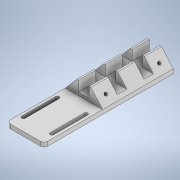
# Autodesk Inventor part: sun2
Saved by Autodesk Inventor 2021 (Build 250183000, 183)
## iProperties
Created: 2021-04-13
Part Number: sun2
Material: 일반
Document SubType Name: Modeling
Designer: Dongyoon
Density: 1 g/cm^3
Appearance: 기본값
Author: Dongyoon
Autodesk Inventor part; units mm, degrees
ref_plane "YZ Plane" through (0, 0, 0) normal (1, 0, 0) x (0, 1, 0)
ref_plane "XZ Plane" through (0, 0, 0) normal (0, 1, 0) x (-1, 0, 0)
ref_plane "XY Plane" through (0, 0, 0) normal (0, 0, 1) x (1, 0, 0)
sketch "스케치1" plane through (0, 0, 0) normal (0, 1, 0) x (-1, 0, 0)
  line L0 (-21.65, 75) -> (21.65, 75)
  line L1 (21.65, 75) -> (21.65, -75)
  line L2 (21.65, -75) -> (-21.65, -75)
  line L3 (-21.65, -75) -> (-21.65, 75)
  line L4 (-21.65, 75) -> (21.65, -75) construction
  line L5 (21.65, 75) -> (-21.65, -75) construction
  line L6 (-21.65, 7) -> (21.65, 7)
  point P0 (0, 0)
  dimension "d0" = 43.3
  dimension "d1" = 150
  dimension "d2" = 68
  constraints: 14 end point, 2 midpoint, 2 parallel, 2 perpendicular, 2 point on line, 1 horizontal
  measures "d0" distance of L1.end L2.end
  measures "d1" distance of L2.end L0.start
  measures "d2" distance between parallel lines of L0 L6
extrude "돌출2" add sketch "스케치1" along normal blind 5 contours L0 L1 L6 L3
extrude "돌출3" add sketch "스케치1" along normal blind 8.5 contours L6 L1 L2 L3
sketch "스케치3" plane through (0, 8.5, 0) normal (0, 1, 0) x (1, 0, 0)
  line L0 (-21.65, -7) -> (21.65, -7) projected
  line L1 (21.65, 75) -> (-21.65, 75) projected
  line L2 (6.1, -7) -> (-6.1, -7)
  line L3 (-6.1, -7) -> (-6.1, 75)
  line L4 (-6.1, 75) -> (6.1, 75)
  line L5 (6.1, 75) -> (6.1, -7)
  line L6 (21.65, -7) -> (21.65, 75) projected
  line L7 (21.65, 75) -> (6.1, 75)
  line L8 (6.1, 75) -> (6.1, -7)
  line L9 (6.1, -7) -> (21.65, -7)
  line L10 (21.65, -7) -> (21.65, 75)
  line L11 (-21.65, 75) -> (-6.1, 75)
  line L12 (-6.1, 75) -> (-6.1, -7)
  line L13 (-6.1, -7) -> (-21.65, -7)
  line L14 (-21.65, -7) -> (-21.65, 75)
  point P0 (0, 0)
  point P1 (-6.1, -7)
  point P2 (6.1, 75)
  dimension "d9" = 12.2
  dimension "d11" = 6.1
  constraints: 24 end point, 6 parallel, 3 horizontal, 3 perpendicular, 2 point on line
  measures "d9" distance between parallel lines of L5 L3
  measures "d11" distance from line of point (0, 0) L5
extrude "돌출4" add sketch "스케치3" along normal blind 12.2 contours L14 L1 L3 L0 | L5 L1 L6 L0
sketch "스케치4" plane through (0, 5, 0) normal (0, 1, 0) x (1, 0, 0)
  line L0 (16.55, -19.1) -> (16.55, -62.7) construction
  line L1 (14.55, -21.1) -> (14.55, -60.7)
  line L2 (18.55, -60.7) -> (18.55, -21.1)
  arc A0 (18.55, -21.1) -> (14.55, -21.1) centre (16.55, -21.1) ccw
  arc A1 (14.55, -60.7) -> (18.55, -60.7) centre (16.55, -60.7) ccw
  line L3 (21.65, -75) -> (21.65, -7) projected
  line L4 (-21.65, -75) -> (21.65, -75) projected
  line L5 (21.65, -7) -> (-21.65, -7) projected
  line L6 (0, -7) -> (0, -75)
  line L7 (-16.55, -19.1) -> (-16.55, -62.7) construction
  line L8 (-14.55, -21.1) -> (-14.55, -60.7)
  line L9 (-18.55, -60.7) -> (-18.55, -21.1)
  arc A2 (-14.55, -21.1) -> (-18.55, -21.1) centre (-16.55, -21.1) ccw
  arc A3 (-18.55, -60.7) -> (-14.55, -60.7) centre (-16.55, -60.7) ccw
  point P0 (0, 0)
  point P1 (16.55, -40.9)
  point P2 (-16.55, -40.9)
  dimension "d14" = 43.6
  dimension "d15" = 3.1
  dimension "d16" = 4
  dimension "d17" = 12.3
  constraints: 18 end point, 12 point on circle, 9 symmetric about line, 4 centre point, 4 point on line, 4 tangent, 3 midpoint, 1 parallel, 1 vertical, 2 other
  measures "d14" distance of L0.start L0.end
  measures "d15" distance between parallel lines of L3 L2
  measures "d16" distance between parallel lines of L2 L1
  measures "d17" distance from line of L4 L0.end
extrude "돌출5" cut sketch "스케치4" against normal through all contours A0 L2 A1 L1 | L8 A3 L9 A2
fillet "모깎기1" radius 4.5 2 edges at (21.65, 2.5, 75) (-21.65, 2.5, 75)
sketch "스케치5" plane through (-21.65, 5, 7) normal (0, 0, 1) x (1, 0, 0)
  line L0 (27.75, 3.5) -> (15.55, 3.5) projected
  line L1 (21.65, 3.5) -> (21.65, 29.9168)
  line L2 (43.3, 0) -> (43.3, 15.7) projected
  line L3 (4.5, 0) -> (38.8, 0) projected
  line L4 (43.3, 15.7) -> (27.75, 15.7)
  line L5 (27.75, 15.7) -> (27.75, 0)
  line L6 (27.75, 0) -> (43.3, 0)
  line L7 (43.3, 0) -> (43.3, 15.7)
  line L8 (43.3, 0) -> (29.75, 15.7)
  line L9 (43.3, 15.7) -> (27.75, 15.7) projected
  line L10 (43.3, -5) -> (38.8, -5) projected
  line L11 (0, 0) -> (0, 15.7)
  line L12 (0, 15.7) -> (15.55, 15.7)
  line L13 (0, 0) -> (0, 15.7)
  line L14 (0, 0) -> (13.55, 15.7)
  point P0 (21.65, -5)
  dimension "d21" = 2
  dimension "d22" = 5
  constraints: 20 end point, 6 symmetric about line, 4 point on line, 2 parallel, 1 horizontal, 1 midpoint, 1 perpendicular, 1 vertical
  measures "d21" distance of L4.end L8.end
  measures "d22" distance from line of L10 L8.start
extrude "돌출6" cut sketch "스케치5" against normal through all contours L8 L4 L2 | L11 L12 L14
sketch "스케치7" plane through (-21.65, 5, -75) normal (-0.7570398, 0.6533688, 0) x (0, 0, 1)
  line L0 (0, 20.7387) -> (82, 20.7387) projected
  line L1 (82, 0) -> (0, 0) projected
  line L2 (82, 20.7387) -> (82, 0) projected
  circle A0 centre (10, 9.7387) radius 1.75
  line L3 (82, 28.2909) -> (82, 0) projected
  line L4 (82, 9.7387) -> (0, 9.7387)
  line L5 (0, 24.5057) -> (0, -3.7852) projected
  line L6 (82, 20.7806) -> (0, 20.7806) projected
  line L7 (41, 20.7806) -> (41, 0)
  circle A1 centre (72, 9.7387) radius 1.75
  dimension "d26" = 3.5
  dimension "d28" = 10
  dimension "d39" = 11
  constraints: 4 end point, 3 point on line, 2 centre point, 2 midpoint, 1 horizontal, 1 symmetric about line, 1 other
  measures "d26" diameter of A0
  measures "d28" distance from line of L5 A0.centre
  measures "d39" distance from line of L0 A0.centre
extrude "돌출7" cut sketch "스케치7" against normal blind 10 contours L4 A0 | A0 L4 | A1 L4 | L4 A1
mirror "미러1" about plane through (0, 0, 0) normal (1, 0, 0) of "돌출7"
sketch "스케치9" plane through (0, 8.5, 0) normal (0, 1, 0) x (1, 0, 0)
  ellipse E0 centre (-15.2871, 3) end of major axis (-15.2871, 1.25) minor radius 1.1434 projected
  ellipse E1 centre (-15.2871, 65) end of major axis (-15.2871, 63.25) minor radius 1.1434 projected
  line L0 (-29.6157, 34) -> (32.1158, 34)
  line L1 (-21.65, -7) -> (-21.65, 75) projected
  line L2 (21.65, 75) -> (21.65, -7) projected
  line L3 (-21.65, 13) -> (21.65, 13)
  line L4 (21.65, 13) -> (21.65, 55)
  line L5 (21.65, 55) -> (-21.65, 55)
  line L6 (-21.65, 55) -> (-21.65, 13)
  line L7 (-21.65, 75) -> (-21.65, -70.5) projected
  line L8 (21.65, -70.5) -> (21.65, 75) projected
  line L9 (-21.65, 24) -> (21.65, 24)
  line L10 (21.65, 24) -> (21.65, 44)
  line L11 (21.65, 44) -> (-21.65, 44)
  line L12 (-21.65, 44) -> (-21.65, 24)
  point P0 (0, 0)
  point P1 (21.65, 13)
  point P2 (-21.65, 44)
  dimension "d32" = 10
  dimension "d33" = 10
  dimension "d36" = 20
  dimension "d38" = 11
  constraints: 18 end point, 4 parallel, 4 point on line, 3 horizontal, 2 perpendicular, 2 other
  measures "d32" distance from line of L3 point (-15.287, 3)
  measures "d33" distance from line of point (-15.287, 65) L5
  measures "d36" distance between parallel lines of L11 L9
  measures "d38" distance between parallel lines of L11 L5
extrude "돌출8" cut sketch "스케치9" along normal through all contours L9 L2 L3 L1 | L1 L5 L2 L11
